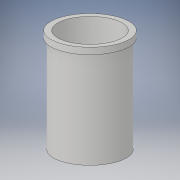
# Autodesk Inventor part: Component 13 (Cylinder Liner)
Saved by Autodesk Inventor 2018 (Build 220112000, 112)
## iProperties
Created: 2023-03-14
Part Number: Component 13 (Cylinder Liner)
Material: Generic
Document SubType Name: Modeling
Designer: Habib Mohamed
Density: 1 g/cm^3
Appearance: Default
Author: Habib Mohamed
Autodesk Inventor part; units mm, degrees
ref_plane "YZ Plane" through (0, 0, 0) normal (1, 0, 0) x (0, 1, 0)
ref_plane "XZ Plane" through (0, 0, 0) normal (0, 1, 0) x (-1, 0, 0)
ref_plane "XY Plane" through (0, 0, 0) normal (0, 0, 1) x (1, 0, 0)
sketch "Sketch1" plane through (0, 0, 0) normal (1, 0, 0) x (0, 1, 0)
  line L0 (0, 0) -> (64.5986, 0) construction
  line L1 (0, -12) -> (40, -12)
  line L2 (40, -12) -> (40, -14.5)
  line L3 (40, -14.5) -> (37.5, -14.5)
  line L4 (37.5, -14.5) -> (37.5, -13.5)
  line L5 (37.5, -13.5) -> (0, -13.5)
  line L6 (0, -13.5) -> (0, -12)
  dimension "d0" = 40
  dimension "d1" = 13.5
  dimension "d2" = 12
  dimension "d3" = 14.5
  dimension "d4" = 2.5
  constraints: 14 end point, 4 perpendicular, 2 horizontal, 1 point on line, 1 vertical
  measures "d0" distance of L1.start L1.end
  measures "d1" distance between parallel lines of L0 L5
  measures "d2" distance between parallel lines of L1 L0
  measures "d3" distance between parallel lines of L3 L0
  measures "d4" distance of L2.end L3.end
revolve "Revolution1" add sketch "Sketch1" angle 360 about axis through (0, 0, 0) along (0, 1, 0)
body "Solid1"
